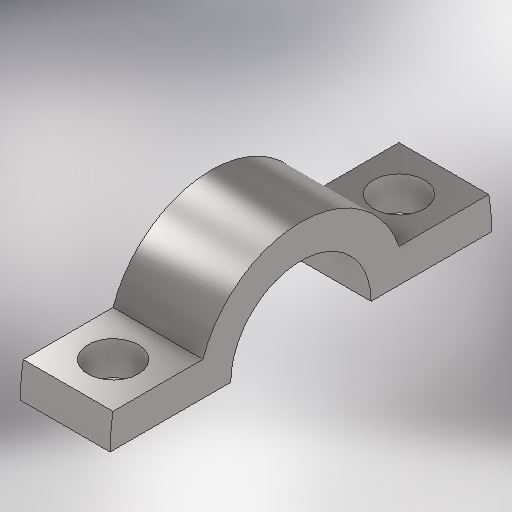
# Autodesk Inventor part: probe-cover-clump
Saved by Autodesk Inventor 2026 (Build 300175050, 175E)
## iProperties
Created: 2025-10-27
Part Number: probe-cover-clump
Material: ステンレス鋼
Document SubType Name: Modeling
Designer: jin20
Density: 8 g/cm^3
Appearance: 半つや出し
Author: jin20
Autodesk Inventor part; units mm, degrees
ref_plane "YZ Plane" through (0, 0, 0) normal (1, 0, 0) x (0, 1, 0)
ref_plane "XZ Plane" through (0, 0, 0) normal (0, 1, 0) x (-1, 0, 0)
ref_plane "XY Plane" through (0, 0, 0) normal (0, 0, 1) x (1, 0, 0)
sketch "スケッチ1" plane through (0, 0, 0) normal (0, 0, 1) x (1, 0, 0)
  line L0 (-5.6, 0) -> (5.6, 0) projected
  line L1 (0, 0) -> (0, 6.25) construction
  line L2 (0, 6.25) -> (-4, 6.25)
  line L3 (-4, 6.25) -> (-4, 17)
  line L4 (-4, 17) -> (0, 17)
  line L5 (0, 6.25) -> (4, 6.25)
  line L6 (4, 6.25) -> (4, 17)
  line L7 (4, 17) -> (0, 17)
  dimension "d32" = 6.25
  dimension "d33" = 4
  dimension "d34" = 10.75
  constraints: 14 end point, 1 horizontal, 1 parallel, 1 perpendicular, 1 vertical
  measures "d32" distance of L1.start L1.end
  measures "d33" distance of L3.end L4.end
  measures "d34" distance of L2.end L3.end
revolve "回転1" add sketch "スケッチ1" angle 180 mid plane about axis through (-10, 0, 0) along (1, 0, 0)
sketch "スケッチ5" plane through (-4, 0, -17) normal (-1, 0, 0) x (0, 0, 1)
  line L0 (17, 0) -> (17, 3) construction
  arc A0 (25.7409, 3) -> (8.2591, 3) centre (17, 0) ccw
  arc A1 (33.7332, 3) -> (0.2668, 3) centre (17, 0) ccw
  line L1 (0.2668, 3) -> (8.2668, 3)
  line L2 (33.7332, 3) -> (25.7332, 3.0224)
  circle A2 centre (17, 0) radius 9.2341
  point P0 (8.2591, 3)
  dimension "d35" = 3
  dimension "d49" = 8
  dimension "d50" = 8
  constraints: 6 end point, 6 point on circle, 2 centre point, 2 coincident, 1 horizontal, 1 vertical, 3 other
  measures "d35" distance of L0.start L0.end
  measures "d49" distance of L1.start L1.end
  measures "d50" distance of L2.start L2.end
extrude "押し出し2" cut sketch "スケッチ5" against normal through all contours A0 L1 A1 L2
sketch "スケッチ7" plane through (-4, 3.0224, 8.7332) normal (0, 1, 0.0028) x (1, 0, 0)
  line L0 (8, -8) -> (0, -8) projected
  line L1 (0, -8) -> (0, 0) projected
  point P0 (4, 8.7247)
  point P1 (4, -4)
  dimension "d51" = 4
  dimension "d52" = 4
  measures "d51" distance from line of L0 point (4, -4)
  measures "d52" distance from line of L1 point (4, -4)
hole "穴4" at (0, 3.0112, 12.7332) direction (0, -1, -0.0028) diameter 4.5 end through all
mirror "ミラー3" about plane through (0, 0, 0) normal (0, 0, 1) of "穴4"
